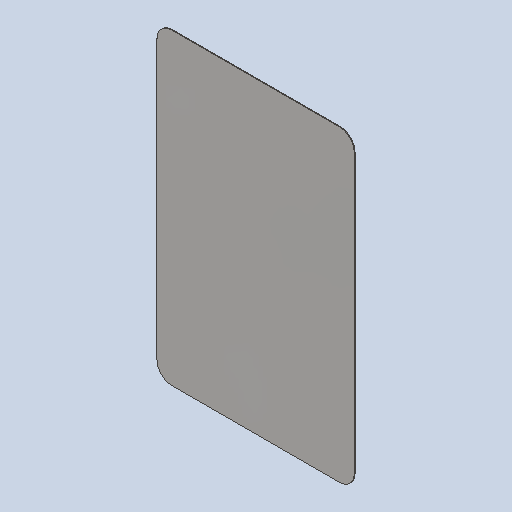
# Autodesk Inventor part: FSI Plate
Saved by Autodesk Inventor 2023 (Build 270158000, 158)
## iProperties
Created: 2022-12-13
Part Number: FSI Plate
Material: ABS Plastic
Document SubType Name: Modeling
Designer: Tanzu
Density: 1.06 g/cm^3
Appearance: Steel - Polished
Mass: 14.7977 g
Surface Area: 561.747 cm^2
Volume: 13.9601 cm^3
Author: Tanzu
Autodesk Inventor part; units mm, degrees
ref_plane "YZ Plane" through (0, 0, 0) normal (1, 0, 0) x (0, 1, 0)
ref_plane "XZ Plane" through (0, 0, 0) normal (0, 1, 0) x (-1, 0, 0)
ref_plane "XY Plane" through (0, 0, 0) normal (0, 0, 1) x (1, 0, 0)
sketch "Sketch1" plane through (0, 0, 0) normal (0, 0, 1) x (1, 0, 0)
  line L0 (-67, 104.5) -> (67, 104.5)
  line L1 (67, 104.5) -> (67, -104.5)
  line L2 (67, -104.5) -> (-67, -104.5)
  line L3 (-67, -104.5) -> (-67, 104.5)
  line L4 (66, 103.5) -> (-66, 103.5)
  line L5 (-66, 103.5) -> (-66, -103.5)
  line L6 (-66, -103.5) -> (66, -103.5)
  line L7 (66, -103.5) -> (66, 103.5)
  point P0 (0, 0)
  point P1 (-67, 0)
  point P2 (0, 104.5)
  dimension "d0" = 134
  dimension "d1" = 209
  dimension "d2" = 1
  constraints: 16 end point, 4 parallel, 2 midpoint, 2 perpendicular, 1 horizontal, 1 horizontal alignment, 1 vertical alignment, 3 other
  measures "d0" distance of L0.start L0.end
  measures "d1" distance of L2.end L0.start
  measures "d2" distance between parallel lines of L0 L4
extrude "Extrusion1" add sketch "Sketch1" against normal blind 0.5 contours L0 L1 L2 L3 | L7 L6 L5 L4
fillet "Fillet1" radius 10 4 edges at (-67, 104.5, -0.25) (67, 104.5, -0.25) (67, -104.5, -0.25) (-67, -104.5, -0.25)
body "Solid1"
